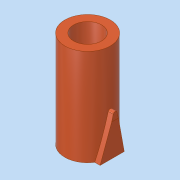
# Autodesk Inventor part: HoleInsertsForBoltsLinkageSection
Saved by Autodesk Inventor 2017 (Build 210142000, 142)
## iProperties
Created: 2018-03-20
Part Number: HoleInsertsForBoltsLinkageSection
Material: ABS Plastic
Document SubType Name: Modeling
Designer: Derek Wider
Density: 1.06 g/cm^3
Appearance: Smooth - Light Orange
Author: Derek Wider
Autodesk Inventor part; units mm, degrees
ref_plane "XZ Plane" through (0, 0, 0) normal (0, 1, 0) x (-1, 0, 0)
ref_plane "XY Plane" through (0, 0, 0) normal (0, 0, 1) x (1, 0, 0)
sketch "Sketch1" plane through (0, 0, 0) normal (0, 1, 0) x (-1, 0, 0)
  circle A0 centre (0, 0) radius 2.9845
  circle A1 centre (0, 0) radius 1.8415
  dimension "d0" = 5.969
  dimension "d1" = 3.683
  constraints: 2 centre point, 2 coincident
  measures "d0" diameter of A0
  measures "d1" diameter of A1
extrude "Extrusion1" add sketch "Sketch1" along normal blind 12.7
ref_plane "Work Plane1" through (2.9845, 0, 0) normal (1, 0, 0) x (0, 1, 0)
sketch "Sketch2" plane through (2.9845, 0, 0) normal (1, 0, 0) x (0, 1, 0)
  line L0 (6.35, 0) -> (0, 1.5875)
  line L1 (0, 1.5875) -> (0, -1.5875)
  line L2 (0, 2.9845) -> (0, -2.9845) projected
  line L3 (6.35, 0) -> (0, -1.5875)
  line L4 (0, -1.5875) -> (0, 0) construction
  line L5 (0, 0) -> (0, 1.5875) construction
  dimension "d4" = 3.175
  dimension "d5" = 6.35
  constraints: 10 end point, 2 collinear, 1 point on line, 1 vertical
  measures "d4" distance of L0.end L1.end
  measures "d5" distance from line of L1 L0.start
extrude "Extrusion2" add sketch "Sketch2" along normal blind 0.635 and the other way blind 0.762
fillet "Fillet1" radius 0.254 1 edges at (3.302, 6.35, 0)
chamfer "Chamfer1" distance 4.572 distance2 0.381 1 edges at (3.6195, 0, 0) measured on face at (3.6195, 0.5, 0)
body "Solid1"
